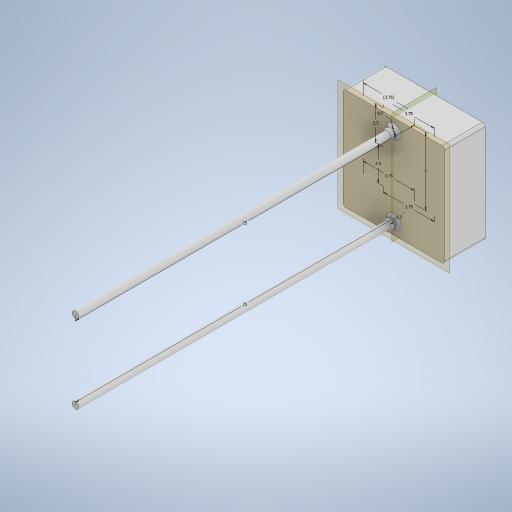
# Autodesk Inventor part: A60
Saved by Autodesk Inventor 2024 (Build 280153000, 153)
## iProperties
Created: 2023-12-15
Part Number: A60
Material: Generic
Document SubType Name: Sheet Metal
Designer: user
Density: 1 g/cm^3
Sheet Metal Rule: Default
Appearance: Default
Author: user
Autodesk Inventor part; units mm, degrees
ref_plane "YZ Plane" through (0, 0, 0) normal (1, 0, 0) x (0, 1, 0)
ref_plane "XZ Plane" through (0, 0, 0) normal (0, 1, 0) x (-1, 0, 0)
ref_plane "XY Plane" through (0, 0, 0) normal (0, 0, 1) x (1, 0, 0)
sketch "Sketch1" plane through (0, 0, 0) normal (0, 0, 1) x (1, 0, 0)
  line L0 (7.3, 7.5) -> (0.2, 7.5)
  line L1 (0, 7.3) -> (0, 0.2)
  line L2 (0.2, 0) -> (7.3, 0)
  line L3 (7.5, 0.2) -> (7.5, 7.3)
  arc A0 (7.5, 7.3) -> (7.3, 7.5) centre (7.3, 7.3) ccw
  arc A1 (0.2, 7.5) -> (0, 7.3) centre (0.2, 7.3) ccw
  arc A2 (0, 0.2) -> (0.2, 0) centre (0.2, 0.2) ccw
  arc A3 (7.3, 0) -> (7.5, 0.2) centre (7.3, 0.2) ccw
  point P0 (0, 0)
  point P1 (0, 7.5)
  point P2 (7.5, 0)
  dimension "d0" = 7.5
  dimension "d1" = 7.5
  dimension "d2" = 0.2
  constraints: 8 end point, 8 point on circle, 8 tangent, 6 point on line, 4 centre point, 3 equal radius, 2 parallel, 1 horizontal, 1 perpendicular
  measures "d0" distance of point (7.5, 0) point (0, 0)
  measures "d1" distance of point (0, 0) point (0, 7.5)
  measures "d2" radius of A0
extrude "Extrusion1" add sketch "Sketch1" along normal mid plane 3
sketch "Sketch3" plane through (0, 0, 0) normal (0, 0, 1) x (1, 0, 0)
  line L0 (0, 7.3) -> (0, 0.2) projected
  line L1 (1.4869, 3.75) -> (1.4869, 1.25)
  line L2 (1.4869, 1.25) -> (5.2369, 1.25)
  line L3 (1.4869, 3.75) -> (1.4869, 6.25)
  line L4 (1.4869, 6.25) -> (5.2369, 6.25)
  line L5 (1.4869, 1.25) -> (0, 1.25)
  line L6 (0, 1.25) -> (3.75, 1.25)
  line L7 (3.75, 1.25) -> (3.75, 6.25)
  line L8 (3.75, 6.25) -> (0, 6.25)
  point P0 (0, 0)
  dimension "d7" = 2.5
  dimension "d8" = 3.75
  dimension "d9" = 2.5
  dimension "d10" = 3.75
  dimension "d11" = 3.75
  dimension "d12" = 5
  dimension "d13" = 3.75
  constraints: 16 end point, 4 point on line, 3 perpendicular, 2 vertical
  measures "d7" distance of L1.start L1.end
  measures "d8" distance of L1.end L2.end
  measures "d9" distance of L1.start L3.end
  measures "d10" distance of L3.end L4.end
  measures "d11" distance of L5.end L6.end
  measures "d12" distance of L6.end L7.end
  measures "d13" distance of L7.end L8.end
ref_plane "Work Plane1" through (3.75, 0.2, 1.5) normal (-1, 0, 0) x (0, 0, 1)
sketch "Sketch4" plane through (3.75, 0.2, 1.5) normal (-1, 0, 0) x (0, 0, 1)
  line L0 (-1.5, 6.4485) -> (23.5, 6.4485)
  line L1 (-1.5, 0.671) -> (23.5, 0.671)
  point P0 (-1.5, -0.2)
  dimension "d15" = 25
  dimension "d17" = 25
  constraints: 4 end point
  measures "d15" distance of L0.start L0.end
  measures "d17" distance of L1.start L1.end
ref_plane "Work Plane2" through (0, 0, 1.5) normal (0, 0, 1) x (1, 0, 0)
sketch "Sketch6" plane through (0, 0, 1.5) normal (0, 0, 1) x (1, 0, 0)
  circle A0 centre (3.7506, 6.6485) radius 0.35
  circle A1 centre (3.7506, 0.8713) radius 0.35
  point P0 (0, 0)
  dimension "d22" = 0.7
  dimension "d27" = 0.7
  constraints: 2 centre point
  measures "d22" diameter of A0
  measures "d27" diameter of A1
extrude "Extrusion3" add sketch "Sketch6" along normal blind 0.5 contours A0
fillet "Fillet3" radius 0.2 2 edges at (3.4006, 6.6485, 1.5) (3.4006, 6.6485, 2)
extrude "Extrusion4" add sketch "Sketch6" along normal blind 0.5 contours A1
fillet "Fillet4" radius 0.2 2 edges at (3.4006, 0.8713, 2) (3.4006, 0.8713, 1.5)
ref_plane "Work Plane3" through (3.7506, 0.8713, 2) normal (0, 0, 1) x (1, 0, 0)
ref_plane "Work Plane4" through (3.7506, 6.6485, 2) normal (0, 0, 1) x (1, 0, 0)
sketch "Sketch7" plane through (3.7506, 0.8713, 2) normal (0, 0, 1) x (1, 0, 0)
  circle A0 centre (0, 0) radius 0.25
  point P0 (-3.7506, -0.8713)
  dimension "d33" = 0.5
  constraints: 1 centre point
  measures "d33" diameter of A0
sweep "Sweep1" add profiles "Sketch7" path "Sketch4" path curves L1
sketch "Sketch8" plane through (3.7506, 6.6485, 2) normal (0, 0, 1) x (1, 0, 0)
  circle A0 centre (0, 0) radius 0.25
  point P0 (-3.7506, -6.6485)
  dimension "d36" = 0.5
  constraints: 1 centre point
  measures "d36" diameter of A0
sweep "Sweep2" add profiles "Sketch8" path "Sketch4" path curves L0
equation "\"BendRadius\" = Thickness"
equation "\"BendReliefWidth\" = Thickness"
equation "\"BendReliefDepth\" = 0.5 * Thickness"
equation "\"CornerReliefSize\" = 4 * Thickness"
equation "\"MinimumRemnant\" = 2 * Thickness"
equation "\"TransitionRadius\" = BendRadius"
equation "\"JacobiRadiusSize\" = BendRadius"
equation "\"GapSize\" = Thickness"
equation "\"Thickness\" = 3.048"
body "Solid1"
